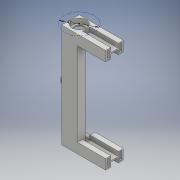
# Autodesk Inventor part: frontAxelHolder 10-24
Saved by Autodesk Inventor 2018 (Build 220112000, 112)
## iProperties
Created: 2019-10-24
Part Number: frontAxelHolder 10-24
Material: Generic
Document SubType Name: Modeling
Designer: Aditya Kendre
Density: 1 g/cm^3
Appearance: Default
Author: Aditya Kendre
## iProperties of the stored document frontAxelHolder 10-24_3DPrint.ipt
Created: 2019-10-24
Part Number: frontAxelHolder 10-24_3DPrint
Material: Generic
Document SubType Name: Modeling
Designer: Aditya Kendre
Density: 1 g/cm^3
Appearance: Default
Author: Aditya Kendre
Autodesk Inventor part; units mm, degrees
ref_plane "YZ Plane" through (0, 0, 0) normal (1, 0, 0) x (0, 1, 0)
ref_plane "XZ Plane" through (0, 0, 0) normal (0, 1, 0) x (-1, 0, 0)
ref_plane "XY Plane" through (0, 0, 0) normal (0, 0, 1) x (1, 0, 0)
sketch "Sketch1" plane through (0, 0, 0) normal (0, 1, 0) x (-1, 0, 0)
  line L0 (0, 0) -> (25, 0)
  line L1 (25, 0) -> (25, -165)
  line L2 (25, -165) -> (0, -165)
  line L3 (0, -165) -> (0, 0)
  dimension "d0" = 25
  dimension "d1" = 165
  constraints: 8 end point, 2 parallel, 1 horizontal, 1 perpendicular
  measures "d0" distance of L1.end L2.end
  measures "d1" distance of L0.end L1.end
extrude "Extrusion1" add sketch "Sketch1" along normal blind 3
sketch "Sketch2" plane through (0, 3, 0) normal (0, 1, 0) x (1, 0, 0)
  line L0 (0, 0) -> (0, 165) projected
  line L1 (-25, 165) -> (-25, 0) projected
  line L2 (0, 0) -> (-25, 0)
  line L3 (-25, 0) -> (-25, 8.5)
  line L4 (-25, 8.5) -> (0, 8.5)
  line L5 (0, 8.5) -> (0, 0)
  line L6 (-25, 165) -> (0, 165)
  line L7 (0, 165) -> (0, 156.5)
  line L8 (0, 156.5) -> (-25, 156.5)
  line L9 (-25, 156.5) -> (-25, 165)
  dimension "d4" = 8.5
  dimension "d5" = 8.5
  constraints: 16 end point, 4 parallel, 2 horizontal, 2 perpendicular, 2 point on line
  measures "d4" distance of L2.end L3.end
  measures "d5" distance of L6.end L7.end
extrude "Extrusion2" add sketch "Sketch2" along normal blind 25 contours L2 L1 L4 L0 | L8 L1 L6 L0
sketch "Sketch3" plane through (-25, 0, 0) normal (0, 0, 1) x (1, 0, 0)
  line L0 (0, 3) -> (0, 28) construction
  line L1 (25, 3) -> (25, 28) construction
  line L2 (0, 28) -> (25, 28) construction
  line L3 (25, 28) -> (25, 3) construction
  line L4 (25, 3) -> (0, 3) construction
  line L5 (0, 3) -> (0, 28) construction
  circle A0 centre (12.5, 15.5) radius 11.375
  point P0 (25, 0)
  dimension "d8" = 25
  dimension "d9" = 22.75
  constraints: 8 end point, 2 parallel, 1 centre point, 1 horizontal, 1 perpendicular
  measures "d8" distance of L2.end L1.start
  measures "d9" diameter of A0
extrude "Extrusion3" cut sketch "Sketch3" against normal blind 7.1
sketch "Sketch4" plane through (-25, 0, 0) normal (0, 0, 1) x (1, 0, 0)
  circle A0 centre (12.5, 15.5) radius 11.375 projected
  circle A1 centre (12.5, 15.5) radius 7.75
  point P0 (25, 0)
  dimension "d12" = 15.5
  constraints: 1 centre point, 1 coincident
  measures "d12" diameter of A1
extrude "Extrusion4" cut sketch "Sketch4" against normal blind 165 contours A1
sketch "Sketch5" plane through (0, 0, -165) normal (0, 0, -1) x (-1, 0, 0)
  circle A0 centre (12.5, 15.5) radius 7.75 projected
  circle A1 centre (12.5, 15.5) radius 11
  point P0 (0, 0)
  constraints: 1 centre point, 1 coincident
extrude "Extrusion5" cut sketch "Sketch5" against normal blind 7.1
sketch "Sketch6" plane through (0, 3, 0) normal (0, 1, 0) x (1, 0, 0)
  line L0 (-25, 156.5) -> (-25, 8.5) projected
  line L1 (-20.25, 8.5) -> (-4.75, 8.5) projected
  line L2 (-25, 156.5) -> (-20, 156.5)
  line L3 (-20, 156.5) -> (-20, 8.5)
  line L4 (-20, 8.5) -> (-25, 8.5)
  line L5 (-25, 8.5) -> (-25, 156.5)
  line L6 (0, 8.5) -> (0, 156.5) projected
  line L7 (-4.75, 156.5) -> (-20.25, 156.5) projected
  line L8 (0, 8.5) -> (-5, 8.5)
  line L9 (-5, 8.5) -> (-5, 156.5)
  line L10 (-5, 156.5) -> (0, 156.5)
  line L11 (0, 156.5) -> (0, 8.5)
  point P0 (0, 0)
  dimension "d17" = 5
  dimension "d18" = 5
  constraints: 16 end point, 4 parallel, 2 horizontal, 2 perpendicular, 2 point on line
  measures "d17" distance of L3.end L4.end
  measures "d18" distance of L9.end L10.end
extrude "Extrusion6" add sketch "Sketch6" along normal blind 10 contours L2 L3 L1 L4 L0 | L7 L10 L6 L8 L1 L9
fillet "Fillet1" radius 2 2 edges at (-5, 13, -82.5) (-20, 13, -82.5)
sketch "Sketch7" plane through (0, 0, 0) normal (1, 0, 0) x (0, 0, -1)
  line L0 (165, 0) -> (0, 0) projected
  line L1 (0, 0) -> (16, 0)
  line L2 (16, 0) -> (16, 8)
  line L3 (16, 8) -> (0, 8)
  line L4 (0, 8) -> (0, 0)
  line L5 (165, 0) -> (149, 0)
  line L6 (149, 0) -> (149, 8)
  line L7 (149, 8) -> (165, 8)
  line L8 (165, 8) -> (165, 0)
  line L9 (0, 28) -> (8.5, 28) projected
  line L10 (0, 28) -> (16, 28)
  line L11 (16, 28) -> (16, 20)
  line L12 (16, 20) -> (0, 20)
  line L13 (0, 20) -> (0, 28)
  line L14 (165, 0) -> (165, 28) projected
  line L15 (165, 28) -> (149, 28)
  line L16 (149, 28) -> (149, 20)
  line L17 (149, 20) -> (165, 20)
  line L18 (165, 20) -> (165, 28)
  dimension "d22" = 16
  dimension "d23" = 8
  dimension "d24" = 16
  dimension "d25" = 16
  dimension "d26" = 8
  constraints: 32 end point, 8 parallel, 4 horizontal, 4 perpendicular, 3 point on line
  measures "d22" distance of L3.end L2.end
  measures "d23" distance of L2.end L1.end
  measures "d24" distance of L6.end L7.end
  measures "d25" distance of L11.end L12.end
  measures "d26" distance of L10.end L11.end
extrude "Extrusion7" add sketch "Sketch7" along normal blind 45
fillet "Fillet2" radius 6 2 edges at (0, 24, -156.5) (0, 24, -8.5)
sketch "Sketch8" plane through (45, 0, 0) normal (1, 0, 0) x (0, 0, -1)
  line L0 (8.5, 20) -> (0, 20) construction
  line L1 (16, 28) -> (16, 20) construction
  line L2 (0, 20) -> (16, 28) construction
  line L3 (0, 0) -> (165, 0) construction
  line L4 (16, 8) -> (16, 0) construction
  line L5 (0, 0) -> (16, 8) construction
  line L6 (150.5, 28) -> (149, 28) construction
  line L7 (165, 8) -> (165, 20) construction
  line L8 (149, 28) -> (165, 20) construction
  line L9 (149, 0) -> (149, 8) construction
  line L10 (149, 8) -> (165, 0) construction
  line L11 (163.125, 22.25) -> (150.875, 22.25)
  line L12 (150.875, 22.25) -> (150.875, 25.75)
  line L13 (150.875, 25.75) -> (163.125, 25.75)
  line L14 (163.125, 25.75) -> (163.125, 22.25)
  line L15 (163.125, 22.25) -> (150.875, 25.75) construction
  line L16 (150.875, 22.25) -> (163.125, 25.75) construction
  line L17 (163.125, 2.25) -> (150.875, 2.25)
  line L18 (150.875, 2.25) -> (150.875, 5.75)
  line L19 (150.875, 5.75) -> (163.125, 5.75)
  line L20 (163.125, 5.75) -> (163.125, 2.25)
  line L21 (163.125, 2.25) -> (150.875, 5.75) construction
  line L22 (150.875, 2.25) -> (163.125, 5.75) construction
  line L23 (14.125, 22.25) -> (1.875, 22.25)
  line L24 (1.875, 22.25) -> (1.875, 25.75)
  line L25 (1.875, 25.75) -> (14.125, 25.75)
  line L26 (14.125, 25.75) -> (14.125, 22.25)
  line L27 (14.125, 22.25) -> (1.875, 25.75) construction
  line L28 (1.875, 22.25) -> (14.125, 25.75) construction
  line L29 (14.125, 2.25) -> (1.875, 2.25)
  line L30 (1.875, 2.25) -> (1.875, 5.75)
  line L31 (1.875, 5.75) -> (14.125, 5.75)
  line L32 (14.125, 5.75) -> (14.125, 2.25)
  line L33 (14.125, 2.25) -> (1.875, 5.75) construction
  line L34 (1.875, 2.25) -> (14.125, 5.75) construction
  point P0 (157, 24)
  point P1 (157, 4)
  point P2 (8, 24)
  point P3 (8, 4)
  dimension "d30" = 12.25
  dimension "d31" = 3.5
  dimension "d32" = 12.25
  dimension "d33" = 3.5
  dimension "d34" = 12.25
  dimension "d35" = 12.25
  dimension "d36" = 3.5
  constraints: 56 end point, 12 midpoint, 8 parallel, 4 horizontal, 4 perpendicular, 1 point on line
  measures "d30" distance of L12.end L13.end
  measures "d31" distance of L11.end L12.end
  measures "d32" distance of L18.end L19.end
  measures "d33" distance of L17.end L18.end
  measures "d34" distance of L24.end L25.end
  measures "d35" distance of L30.end L31.end
  measures "d36" distance of L29.end L30.end
extrude "Extrusion8" cut sketch "Sketch8" against normal blind 40
sketch "Sketch9" plane through (0, 8, 0) normal (0, 1, 0) x (1, 0, 0)
  line L0 (0, 0) -> (0, 16) construction
  line L1 (0, 8) -> (0, 9) construction
  line L2 (45, 1.875) -> (45, 14.125) construction
  line L3 (0, 9) -> (45, 9) construction
  line L4 (45, 9) -> (45, 7) construction
  line L5 (45, 7) -> (0, 7) construction
  line L6 (0, 7) -> (0, 9) construction
  line L7 (0, 9) -> (45, 9)
  line L8 (45, 9) -> (45, 7)
  line L9 (45, 7) -> (0, 7)
  line L10 (0, 7) -> (0, 9)
  line L11 (0, 149) -> (0, 165) construction
  line L12 (0, 149) -> (0, 157) construction
  line L13 (0, 157) -> (0, 158) construction
  line L14 (45, 165) -> (45, 149) projected
  line L15 (0, 158) -> (45, 158)
  line L16 (45, 158) -> (45, 156)
  line L17 (45, 156) -> (0, 156)
  line L18 (0, 156) -> (0, 158)
  dimension "d39" = 1
  dimension "d40" = 2
  dimension "d41" = 8
  dimension "d42" = 1
  dimension "d43" = 2
  constraints: 30 end point, 6 parallel, 4 point on line, 3 horizontal, 3 perpendicular, 1 midpoint, 1 vertical
  measures "d39" distance of L1.start L1.end
  measures "d40" distance of L3.end L4.end
  measures "d41" distance of L11.start L12.end
  measures "d42" distance of L12.end L13.end
  measures "d43" distance of L15.end L16.end
extrude "Extrusion9" add sketch "Sketch9" along normal blind 12
fillet "Fillet3" radius 6 2 edges at (0, 16.5, -156.5) (0, 16.5, -8.5)
sketch "Sketch10" plane through (-25, 0, -165) normal (-1, 0, 0) x (0, 0, 1)
  line L0 (165, 0) -> (0, 0) construction
  line L1 (82.5, 0) -> (82.5, 6) construction
  line L2 (156.5, 13) -> (8.5, 13) construction
  line L3 (82.5, 6) -> (86.5, 6) construction
  line L4 (86.5, 6) -> (86.5, 13) construction
  line L5 (86.5, 13) -> (82.5, 13) construction
  line L6 (82.5, 13) -> (82.5, 6) construction
  line L7 (86.5, 6) -> (78.5, 6)
  line L8 (78.5, 6) -> (78.5, 13)
  line L9 (78.5, 13) -> (86.5, 13)
  line L10 (86.5, 13) -> (86.5, 6)
  dimension "d47" = 6
  dimension "d48" = 4
  dimension "d49" = 8
  constraints: 18 end point, 4 parallel, 2 horizontal, 2 perpendicular, 2 point on line, 1 midpoint, 1 vertical
  measures "d47" distance of L1.start L1.end
  measures "d48" distance of L5.end L4.end
  measures "d49" distance of L8.end L9.end
extrude "Extrusion10" add sketch "Sketch10" along normal blind 6.5
sketch "Sketch11" plane through (0, 13, 0) normal (0, 1, 0) x (1, 0, 0)
  line L0 (-25, 156.5) -> (-25, 86.5) construction
  line L1 (-31.5, 78.5) -> (-31.5, 86.5) construction
  line L2 (-25, 86.5) -> (-31.5, 78.5) construction
  circle A0 centre (-28.25, 82.5) radius 3.175
  point P0 (0, 0)
  dimension "d52" = 6.35
  constraints: 2 end point, 1 centre point, 1 midpoint
  measures "d52" diameter of A0
extrude "Extrusion11" cut sketch "Sketch11" against normal blind 8
fillet "Fillet4" radius 6.5 2 edges at (-25, 9.5, -86.5) (-25, 9.5, -78.5)
sketch "Sketch12" plane through (-25, 0, 0) normal (0, 0, 1) x (1, 0, 0)
  circle A0 centre (12.5, 15.5) radius 7.75 construction
  circle A1 centre (12.5, 15.5) radius 23.5 construction
  point P0 (25, 0)
  dimension "d56" = 47
  constraints: 1 centre point, 1 coincident
  measures "d56" diameter of A1
sketch "Sketch13" plane through (0, 13, 0) normal (0, 1, 0) x (1, 0, 0)
  line L0 (-31.5, 86.5) -> (-31.5, 78.5) projected
  line L1 (-31.5, 86.5) -> (-32.5, 86.5)
  line L2 (-32.5, 86.5) -> (-32.5, 78.5)
  line L3 (-32.5, 78.5) -> (-31.5, 78.5)
  line L4 (-31.5, 78.5) -> (-31.5, 86.5)
  point P0 (0, 0)
  dimension "d57" = 1
  constraints: 8 end point, 2 parallel, 1 horizontal, 1 perpendicular
  measures "d57" distance of L3.end L2.end
extrude "Extrusion12" add sketch "Sketch13" against normal blind 7
sketch "Sketch14" plane through (-25, 0, -165) normal (0, 0, -1) x (-1, 0, 0)
  circle A0 centre (-12.5, 15.5) radius 11.375 projected
  circle A1 centre (-12.5, 15.5) radius 11.375
  point P0 (-25, 0)
  constraints: 1 centre point, 1 coincident
extrude "Extrusion13" cut sketch "Sketch14" against normal blind 7.1
body "Solid1"
